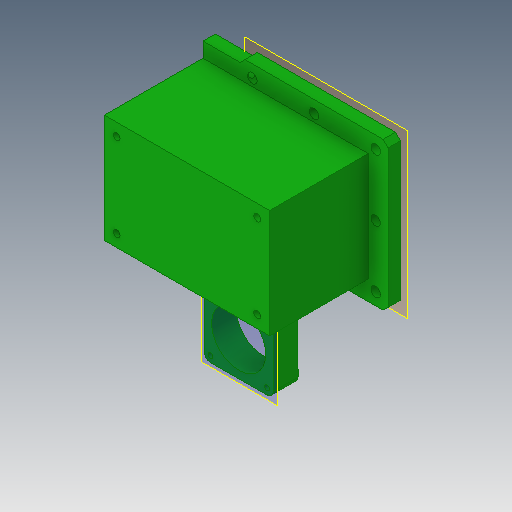
# Autodesk Inventor part: cellSTORM_v5_cellphonestage
Saved by Autodesk Inventor 2019.4 (Build 234330000, 330)
## iProperties
Created: 2020-04-25
Part Number: cellSTORM_v5_cellphonestage
Material: Generic
Document SubType Name: Modeling
Designer: diederichbenedict
Density: 1 g/cm^3
Appearance: Dark Green
Author: diederichbenedict
Autodesk Inventor part; units mm, degrees
ref_plane "YZ Plane" through (0, 0, 0) normal (1, 0, 0) x (0, 1, 0)
ref_plane "XZ Plane" through (0, 0, 0) normal (0, 1, 0) x (-1, 0, 0)
ref_plane "XY Plane" through (0, 0, 0) normal (0, 0, 1) x (1, 0, 0)
ref_plane "Work Plane1" through (0, 0, 0) normal (0, 0, 1) x (1, 0, 0)
sketch "Sketch1" plane through (0, 0, 0) normal (0, 0, 1) x (1, 0, 0)
  circle A0 centre (25, 25) radius 1.95 projected
  circle A1 centre (25, 0) radius 1.95 projected
  circle A2 centre (0, 25) radius 1.95 projected
  circle A3 centre (-25, 0) radius 1.95 projected
  circle A4 centre (-25, -25) radius 1.95 projected
  circle A5 centre (25, 25) radius 1.95 projected
  circle A6 centre (25, -25) radius 1.95 projected
  circle A7 centre (-25, 25) radius 1.95 projected
  circle A8 centre (25, 0) radius 1.95 projected
  circle A9 centre (0, -25) radius 1.95 projected
  line L0 (-28, 30) -> (-30, 28) projected
  line L1 (-30, 28) -> (-30, -28) projected
  line L2 (-30, -28) -> (-28, -30) projected
  line L3 (-28, -30) -> (28, -30) projected
  line L4 (28, -30) -> (30, -28) projected
  line L5 (30, -28) -> (30, 28) projected
  line L6 (30, 28) -> (28, 30) projected
  line L7 (28, 30) -> (-28, 30) projected
  point P0 (0, 0)
extrude "Extrusion1" add sketch "Sketch1" along normal blind 5
sketch "Sketch2" plane through (0, 0, 5) normal (0, 0, 1) x (1, 0, 0)
  circle A0 centre (0, -25) radius 1.95 projected
  circle A1 centre (-25, 25) radius 1.95 projected
  circle A2 centre (25, -25) radius 1.95 projected
  circle A3 centre (-25, -25) radius 1.95 projected
  circle A4 centre (-25, 0) radius 1.95 projected
  circle A5 centre (0, 25) radius 1.95 projected
  circle A6 centre (25, 0) radius 1.95 projected
  circle A7 centre (25, 25) radius 1.95 projected
  line L0 (-28, 30) -> (-30, 28) projected
  line L1 (-30, 28) -> (-30, -28) projected
  line L2 (-30, -28) -> (-28, -30) projected
  line L3 (-28, -30) -> (28, -30) projected
  line L4 (28, -30) -> (30, -28) projected
  line L5 (30, -28) -> (30, 28) projected
  line L6 (30, 28) -> (28, 30) projected
  line L7 (28, 30) -> (-28, 30) projected
  line L8 (-30, 28) -> (-30, -28) projected
  line L9 (-30, -22) -> (22, -22)
  line L10 (22, -22) -> (22, 22)
  line L11 (22, 22) -> (-30, 22)
  line L12 (-30, 22) -> (-30, -22)
  point P0 (0, 0)
  dimension "d2" = 8
  dimension "d3" = 8
  dimension "d4" = 8
  constraints: 8 end point, 2 parallel, 1 horizontal, 1 perpendicular, 1 point on line
  measures "d2" distance between parallel lines of L9 L3
  measures "d3" distance between parallel lines of L7 L11
  measures "d4" distance between parallel lines of L5 L10
ref_plane "Work Plane2" through (-93.15, -42.6288, 31.9788) normal (0, 0, -1) x (0, 1, 0)
extrude "Extrusion2" add sketch "Sketch2" along normal blind 40 contours A4 | L11 L10 L9 L1
sketch "Sketch3" plane through (-30, -28, 0) normal (-1, 0, 0) x (0, 0, 1)
  line L0 (0, 56) -> (0, 0) projected
  line L1 (0, 0) -> (5, 0) projected
  line L2 (5, 6) -> (5, 0) projected
  line L3 (5, 6) -> (45, 6) projected
  line L4 (5, 50) -> (45, 50) projected
  line L5 (5, 56) -> (5, 50) projected
  line L6 (0, 56) -> (5, 56) projected
  line L7 (45, 50) -> (45, 6) projected
  point P0 (0, 28)
extrude "Extrusion3" add sketch "Sketch3" along normal blind 10
sketch "Sketch4" plane through (22, -22, 0) normal (0, 0, 1) x (1, 0, 0)
  line L0 (-62, 0) -> (0, 0) projected
  line L1 (0, 44) -> (-62, 44) projected
  line L2 (-62, 0) -> (-62, 44) projected
  arc A0 (-111.65, 45.2512) -> (-115.15, 41.7512) centre (-111.65, 41.7512) ccw projected
  line L3 (-115.15, -17.1288) -> (-115.15, 41.7512) projected
  arc A1 (-115.15, -17.1288) -> (-111.65, -20.6288) centre (-111.65, -17.1288) ccw projected
  line L4 (28.35, -20.6288) -> (-111.65, -20.6288) projected
  arc A2 (28.35, -20.6288) -> (31.85, -17.1288) centre (28.35, -17.1288) ccw projected
  line L5 (31.85, 41.7512) -> (31.85, -17.1288) projected
  arc A3 (31.85, 41.7512) -> (28.35, 45.2512) centre (28.35, 41.7512) ccw projected
  line L6 (-111.65, 45.2512) -> (28.35, 45.2512) projected
  line L7 (0, 0) -> (0, 44) projected
  line L8 (-62, 44) -> (0, 44)
  line L9 (0, 44) -> (0, 0)
  line L10 (0, 0) -> (-62, 0)
  line L11 (-62, 0) -> (-62, 44)
  line L12 (-5, 39) -> (-57, 39)
  line L13 (-57, 39) -> (-57, 5)
  line L14 (-57, 5) -> (-5, 5)
  line L15 (-5, 5) -> (-5, 39)
  point P0 (-22, 22)
  dimension "d9" = 5
  constraints: 16 end point, 4 parallel, 2 perpendicular, 1 horizontal, 3 other
  measures "d9" distance between parallel lines of L8 L12
extrude "Extrusion4" cut sketch "Sketch4" along normal blind 40 contours L15 L14 L13 L12
sketch "Sketch6" plane through (-40, -28, 0) normal (-1, 0, 0) x (0, 0, 1)
  line L0 (0, 56) -> (0, 0) projected
  line L1 (0, 0) -> (5, 0) projected
  line L2 (5, 0) -> (5, 6) projected
  line L3 (5, 6) -> (45, 6) projected
  line L4 (45, 50) -> (5, 50) projected
  line L5 (5, 50) -> (5, 56) projected
  line L6 (5, 56) -> (0, 56) projected
  line L7 (45, 6) -> (45, 50) projected
  point P0 (0, 28)
extrude "Extrusion6" add sketch "Sketch6" along normal blind 5
sketch "Sketch7" plane through (-45, -28, 0) normal (-1, 0, 0) x (0, 0, 1)
  circle A0 centre (41, 25.7717) radius 1.45 projected
  circle A1 centre (23.9, 21.2512) radius 1.45 projected
  circle A2 centre (3.3174, 32.2512) radius 1.45 projected
  circle A3 centre (3.3174, 53) radius 1.45 projected
  line L0 (40, 45) -> (40, 11) projected
  circle A4 centre (41, 8.1883) radius 1.45 projected
  circle A5 centre (4.9143, 21.2512) radius 1.45 projected
  circle A6 centre (23.9337, 3.5995) radius 1.45 projected
  circle A7 centre (41, 25.7717) radius 1.45 projected
  circle A8 centre (41.0502, 56) radius 1.45 projected
  circle A9 centre (41, 0.7395) radius 1.45 projected
  circle A10 centre (23.9, 21.2512) radius 1.45 projected
  circle A11 centre (23.9, 13.4229) radius 1.45 projected
  circle A12 centre (41, 43.0063) radius 1.45 projected
  line L1 (37.1004, -11.7636) -> (45, -11.7636) projected
  line L2 (45, -11.7636) -> (45, 58) projected
  line L3 (26.9, 58) -> (26.9, 25.2512) projected
  line L4 (26.9, 25.2512) -> (-10.2763, 25.2512) projected
  line L5 (-10.2763, 25.2512) -> (37.1004, -11.7636) projected
  line L6 (45, 58) -> (26.9, 58) projected
  point P0 (0, 28)
  point P1 (4.6577, 21.4172)
hole "Hole1" at (-45, 15.0063, 41) at (-45, -2.2283, 41) at (-45, -19.8117, 41) at (-45, -14.5771, 23.9) at (-45, -6.7488, 23.9) at (-45, 4.2512, 3.3174) at (-45, 25, 3.3174) at (-45, -6.7488, 4.9143) direction (1, 0, 0) diameter 2.9 depth 20 tip angle 118
pattern_linear "Rectangular Pattern1" count 4 spacing 4 along (0, 0, -1) of "Hole1"
ref_plane "Arbeitsebene3" through (-16.8987, -56.0499, 18.5) normal (0, 0, -1) x (1, 0, 0)
sketch "Skizze8" plane through (-16.8987, -56.0499, 18.5) normal (0, 0, -1) x (1, 0, 0)
  line L0 (-11.7173, -14.1596) -> (11.2824, -14.2743)
  line L1 (-11.7173, -14.1596) -> (11.2824, -14.2743)
  circle A0 centre (11.4094, 11.2112) radius 1.025
  arc A1 (13.9094, 11.1987) -> (11.4218, 13.7112) centre (11.4094, 11.2112) ccw
  circle A2 centre (11.2948, -11.7885) radius 1.025
  line L2 (13.9094, 11.1987) -> (13.7947, -11.801)
  arc A3 (13.9094, 11.1987) -> (11.4218, 13.7112) centre (11.4094, 11.2112) ccw
  line L3 (-11.5779, 13.8258) -> (11.4218, 13.7112)
  arc A4 (-11.5779, 13.8258) -> (-14.0903, 11.3383) centre (-11.5903, 11.3258) ccw
  line L4 (-14.2049, -11.6614) -> (-14.0903, 11.3383)
  arc A5 (-14.2049, -11.6614) -> (-11.7174, -14.1739) centre (-11.7049, -11.6739) ccw
  line L5 (11.2823, -14.2885) -> (-11.7174, -14.1739)
  arc A6 (11.2823, -14.2885) -> (13.7947, -11.801) centre (11.2948, -11.7885) ccw
  circle A7 centre (-0.1478, -0.2313) radius 11
  circle A8 centre (-11.5903, 11.3258) radius 1.025
  circle A9 centre (11.4094, 11.2112) radius 1.025
  circle A10 centre (11.2948, -11.7885) radius 1.025
  circle A11 centre (-11.7049, -11.6739) radius 1.025
  line L6 (38.8987, -34.0499) -> (-28.1013, -34.0499)
  line L7 (38.8987, -34.0499) -> (-28.1013, -34.0499)
  line L8 (-14, -14) -> (13.7838, -14)
  line L9 (13.7838, -14) -> (13.7838, -34.0499)
  line L10 (13.7838, -34.0499) -> (-14, -34.0499)
  line L11 (-14, -34.0499) -> (-14, -14)
  line L12 (-14, -14) -> (-28.1013, -34.0499)
  line L13 (38.8987, -34.0499) -> (-28.1013, -34.0499)
  line L14 (-14, -34.0499) -> (-28.1013, -34.0499)
  line L15 (-28.1013, -34.0499) -> (-14, -14)
  line L16 (-14, -14) -> (-14.1998, -10.6365)
  line L17 (13.7838, -14) -> (13.7947, -11.801)
  point P0 (16.8987, -56.0499)
extrude "Extrusion7" add sketch "Skizze8" along normal blind 10 contours L2 A6 L8 A5 L16 L4 A4 L3 A1 | L17 L8 A6 | L8 L9 L6 L11 A5 L5 A6 | A6 L5 A5 L8 | L8 L16 A5 | L11 L6 L12
sketch "Skizze9" plane through (-2.9893, -67.2486, 18.5) normal (0.9999876, 0.004983, 0) x (0, 0, -1)
  line L0 (0, 25.1991) -> (0, 0) projected
  line L1 (0, 0) -> (10, 0) projected
  line L2 (10, 25.1991) -> (10, 0) projected
  line L3 (18.5, 39.0838) -> (18.5, 95.0831) projected
  line L4 (18.5, 95.0831) -> (13.5, 95.0831) projected
  line L5 (13.5, 39.0838) -> (13.5, 95.0831) projected
  line L6 (18.5, 39.0838) -> (13.5, 39.0838) projected
  line L7 (18.5, 37.0937) -> (18.5, 39.0838) projected
  line L8 (18.5, 39.0838) -> (13.5, 39.0838) projected
  line L9 (13.5, 37.0937) -> (13.5, 39.0838) projected
  line L10 (18.5, 37.0937) -> (13.5, 37.0937) projected
  line L11 (18.5, 37.0937) -> (10, 28.5937)
  line L12 (10, 45.5499) -> (10, 0) projected
  line L13 (18.5, 37.0937) -> (30.5208, 37.0937) construction
  line L14 (10, 28.5937) -> (10, 45.5499)
  line L15 (10, 45.5499) -> (10, 28.5937)
  line L16 (10, 45.5499) -> (18.5, 45.5499)
  line L17 (18.5, 59.583) -> (18.5, 39.0838) projected
  line L18 (18.5, 37.0937) -> (18.5, 45.5499)
  line L19 (18.5, 44.3078) -> (18.5, 40.4078) projected
  line L20 (0, 25.1991) -> (10, 25.1991) projected
  point P0 (18.5, 67.2329)
  dimension "d28" = 135
  constraints: 12 end point, 3 collinear, 2 point on line, 1 equal length, 1 horizontal, 1 perpendicular
  measures "d28" angle of L11 L13
extrude "Extrusion8" add sketch "Skizze9" against normal up to surface contours L6 L5 L16 L3 | L9 L10 L11 L12 L16 L5 surface through (-30.8987, -42.0499, 18.5) normal (-0.8179572, -0.5752791, 0)
sketch "Skizze10" plane through (0, 0, 5) normal (0, 0, 1) x (1, 0, 0)
  circle A0 centre (-25, -25) radius 1.95 projected
  point P0 (0, 0)
extrude "Extrusion9" cut sketch "Skizze10" along normal through all both and the other way through all
sketch "Skizze11" plane through (0, 0, 45) normal (0, 0, 1) x (1, 0, 0)
  line L0 (22, -22) -> (-45, -22) projected
  line L1 (22, -22) -> (22, 22) projected
  line L2 (22, 22) -> (-45, 22) projected
  line L3 (-45, -22) -> (-45, 22) projected
  line L4 (-40, 17) -> (17, 17)
  line L5 (17, 17) -> (17, -17)
  line L6 (17, -17) -> (-40, -17)
  line L7 (-40, -17) -> (-40, 17)
  point P0 (0, 0)
  dimension "d33" = 5
  constraints: 8 end point, 3 other
  measures "d33" distance between parallel lines of L2 L4
hole "Bohrung2" at (-40, 17, 45) at (-40, -17, 45) at (17, -17, 45) at (17, 17, 45) direction (0, 0, -1) diameter 2.8 depth 12 tip angle 118
body "Solid1"
